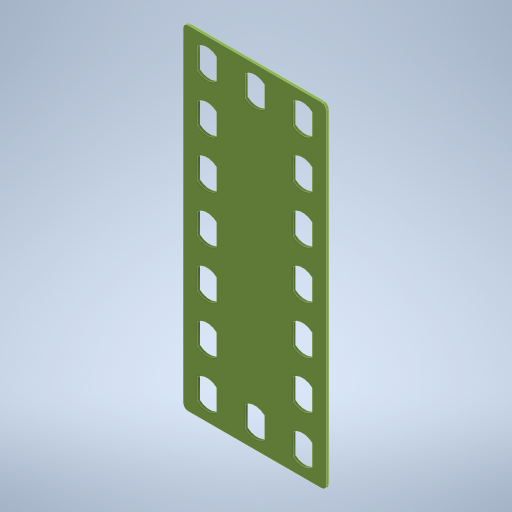
# Autodesk Inventor part: 1018
Saved by Autodesk Inventor 2024 (Build 280153000, 153)
## iProperties
Created: 2024-09-20
Part Number: 1018
Material: Všeobecné
Document SubType Name: Modeling
Designer: Student
Density: 1 g/cm^3
Appearance: Olivově zelená
Author: Student
Autodesk Inventor part; units mm, degrees
ref_plane "YZ Plane" through (0, 0, 0) normal (1, 0, 0) x (0, 1, 0)
ref_plane "XZ Plane" through (0, 0, 0) normal (0, 1, 0) x (-1, 0, 0)
ref_plane "XY Plane" through (0, 0, 0) normal (0, 0, 1) x (1, 0, 0)
sketch "Náčrt1" plane through (0, 0, 0) normal (0, 0, 1) x (1, 0, 0)
  line L0 (-20, 10) -> (10, 10)
  line L1 (10, 10) -> (10, -60)
  line L2 (10, -60) -> (-20, -60)
  line L3 (-20, -60) -> (-20, 10)
  point P0 (0, 0)
  dimension "d0" = 70
  dimension "d1" = 30
  dimension "d2" = 10
  dimension "d3" = 10
  constraints: 8 end point, 2 parallel, 1 horizontal, 1 perpendicular
  measures "d0" distance between parallel lines of L2 L0
  measures "d1" distance between parallel lines of L3 L1
  measures "d2" distance from line of L1 point (0, 0)
  measures "d3" distance from line of L0 point (0, 0)
extrude "Vysunutí1" add sketch "Náčrt1" along normal blind 0.5
fillet "Zaoblení1" radius 1 1 edges at (10, 10, 0.25)
fillet "Zaoblení2" radius 1 2 edges at (-20, 10, 0.25) (-20, -60, 0.25)
fillet "Zaoblení3" radius 1 1 edges at (10, -60, 0.25)
sketch "Náčrt3" plane through (0, 0, 0.5) normal (0, 0, 1) x (1, 0, 0)
  line L0 (7, -52.7639) -> (7, -57.2361)
  line L1 (3, -52.7639) -> (3, -57.2361)
  arc A0 (7, -52.7639) -> (3, -52.7639) centre (5, -55) ccw
  arc A1 (3, -57.2361) -> (7, -57.2361) centre (5, -55) ccw
  line L2 (10, -59) -> (10, 9) projected
  line L3 (-19, -60) -> (9, -60) projected
  point P0 (0, 0)
  point P1 (3, -57.229)
  point P2 (5, -58)
  point P3 (5, -52)
  dimension "d24" = 2
  dimension "d25" = 4
  dimension "d26" = 5
  dimension "d27" = 5
  dimension "d28" = 3
  dimension "d29" = 3
  constraints: 6 point on circle, 4 end point, 2 centre point, 1 point on line
  measures "d24" distance from line of A0.centre L0
  measures "d25" distance from line of point (3, -57.229) L0
  measures "d26" distance from line of L2 A0.centre
  measures "d27" distance from line of L3 A0.centre
  measures "d28" distance of A0.centre point (5, -58)
  measures "d29" distance of A0.centre point (5, -52)
extrude "Vysunutí3" cut sketch "Náčrt3" against normal blind 10
pattern_linear "Obdélníkové pole2" count 7 spacing 10 along (-1, 0, 0) of "Vysunutí3"
pattern_linear "Obdélníkové pole3" count 10 spacing 10 along (0, 1, 0) of "Vysunutí3"
sketch "Náčrt4" plane through (0, 0, 0.5) normal (0, 0, 1) x (1, 0, 0)
  line L0 (-13, 7.2361) -> (-13, 2.7639)
  line L1 (-17, 7.2361) -> (-17, 2.7639)
  arc A0 (-13, 7.2361) -> (-17, 7.2361) centre (-15, 5) ccw
  arc A1 (-17, 2.7639) -> (-13, 2.7639) centre (-15, 5) ccw
  line L2 (9, 10) -> (-19, 10) projected
  line L3 (-20, 9) -> (-20, -59) projected
  point P0 (0, 0)
  point P1 (-17, 2.771)
  point P2 (-15, 2)
  point P3 (-15, 8)
  dimension "d38" = 2
  dimension "d39" = 4
  dimension "d40" = 3
  dimension "d41" = 3
  dimension "d42" = 5
  dimension "d43" = 5
  constraints: 6 point on circle, 4 end point, 2 centre point, 1 point on line
  measures "d38" distance from line of A0.centre L0
  measures "d39" distance from line of point (-17, 2.771) L0
  measures "d40" distance of A0.centre point (-15, 2)
  measures "d41" distance of A0.centre point (-15, 8)
  measures "d42" distance from line of L2 A0.centre
  measures "d43" distance from line of L3 A0.centre
extrude "Vysunutí4" cut sketch "Náčrt4" against normal blind 10
pattern_linear "Obdélníkové pole4" count 9 spacing 10 along (0, -1, 0) of "Vysunutí4"
pattern_linear "Obdélníkové pole5" count 2 spacing 10 along (1, 0, 0) of "Vysunutí4"
